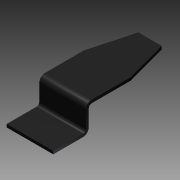
# Autodesk Inventor part: ASAP_Top_Fixture_Handle_New
Saved by Autodesk Inventor 2011 SP2 (Build 150309200, 309)
## iProperties
Created: 2011-11-18
Part Number: ASAP_Top_Fixture_Handle_New
Material: Default
Document SubType Name: Sheet Metal
Designer: sungwook
Density: 1 g/cm^3
Sheet Metal Rule: Default_mm
Author: sungwook
Autodesk Inventor part; units mm, degrees
ref_plane "YZ Plane" through (0, 0, 0) normal (1, 0, 0) x (0, 1, 0)
ref_plane "XZ Plane" through (0, 0, 0) normal (0, 1, 0) x (-1, 0, 0)
ref_plane "XY Plane" through (0, 0, 0) normal (0, 0, 1) x (1, 0, 0)
sketch "Sketch1" plane through (0, 0, 0) normal (0, 0, 1) x (1, 0, 0)
  line L0 (-4, 7.5) -> (4, 7.5)
  line L1 (4, 7.5) -> (4, -7.5)
  line L2 (4, -7.5) -> (-4, -7.5)
  line L3 (-4, -7.5) -> (-4, 7.5)
  line L4 (-2, 7.5) -> (-4, 0.18)
  line L5 (0, -10.5) -> (0, 10.5)
  line L6 (2, 7.5) -> (4, 0.18)
  point P0 (0, 0)
  point P1 (0, 7.5)
  point P2 (-4, 0)
  dimension "d0" = 8
  dimension "d1" = 15
  dimension "d2" = 7.32
  dimension "d3" = 2
  dimension "d4" = 7.32
  dimension "d5" = 4
  measures "d0" distance between parallel lines of L1 L3
  measures "d1" distance between parallel lines of L2 L0
  measures "d2" vertical distance of L4.end L4.start
  measures "d3" distance of point (0, 7.5) L4.start
  measures "d4" vertical distance of L6.end L6.start
  measures "d5" distance of L6.start L4.start
extrude "Plate1" add sketch "Sketch1" along normal blind 0.5 contours L0 L5 L2 L3 L4 | L0 L6 L1 L2 L5
sketch "Sketch2" plane through (-4, -7, 0.5) normal (0, -1, 0) x (1, 0, 0)
  line L0 (8, 0) -> (0, 0)
  line L1 (0, 0) -> (0, -4.8)
  line L2 (0, -4.8) -> (8, -4.8)
  line L3 (8, -4.8) -> (8, 0)
  constraints: 4 end point, 4 other
edge flange "Flange1" height 4.8 angle 90 thickness 0.5 bend radius 0.5 thickness toward (0, -1, 0) relief straight relief width 0.5 relief depth 0.25 edges at (0, -7.5, 0) wall of the first edge with corners at (4, -7, 0.5) (-4, -7, 0.5) (-4, -7, -4.3) (4, -7, -4.3)
bend "Bend1"
corner "Corner1"
sketch "Sketch3" plane through (4, -7, -3.8) normal (0, 0, -1) x (-1, 0, 0)
  line L0 (8, 0) -> (0, 0)
  line L1 (0, 0) -> (0, -6.095)
  line L2 (0, -6.095) -> (8, -6.095)
  line L3 (8, -6.095) -> (8, 0)
  constraints: 4 end point, 4 other
edge flange "Flange2" height 6.095 angle 90 thickness 0.5 bend radius 0.5 thickness toward (0, 0, -1) relief straight relief width 0.5 relief depth 0.25 edges at (0, -7.5, -4.3) wall of the first edge with corners at (-4, -7, -3.8) (4, -7, -3.8) (4, -13.095, -3.8) (-4, -13.095, -3.8)
bend "Bend2"
corner "Corner2"
equation "\"d7\" = BendReliefWidth"
equation "\"d8\" = BendReliefDepth"
equation "\"d9\" = MinimumRemnant"
equation "\"d10\" = BendRadius"
equation "\"d13\" = BendRadius"
equation "\"d14\" = CornerReliefSize"
equation "\"d15\" = GapSize"
equation "\"d16\" = JacobiRadiusSize"
equation "\"d17\" = BendReliefWidth"
equation "\"d18\" = BendReliefDepth"
equation "\"d19\" = MinimumRemnant"
equation "\"d20\" = BendRadius"
equation "\"d23\" = BendRadius"
equation "\"d24\" = CornerReliefSize"
equation "\"d25\" = GapSize"
equation "\"d26\" = JacobiRadiusSize"
equation "\"BendRadius\" = Thickness"
equation "\"BendReliefWidth\" = Thickness"
equation "\"BendReliefDepth\" = 0.5 * Thickness"
equation "\"CornerReliefSize\" = 4 * Thickness"
equation "\"MinimumRemnant\" = 2 * Thickness"
equation "\"TransitionRadius\" = BendRadius"
equation "\"JacobiRadiusSize\" = BendRadius"
equation "\"GapSize\" = Thickness"
equation "\"d6\" = BendRadius"
equation "\"Thickness\" = 0.5"
body "Solid1"
